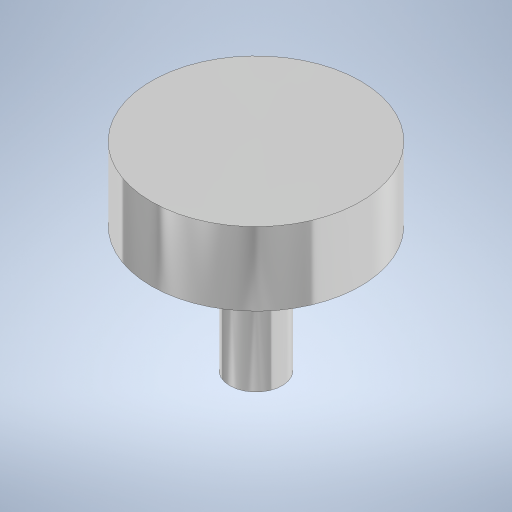
# Autodesk Inventor part: micromanipulator_knob
Saved by Autodesk Inventor 2024 (Build 280153000, 153)
## iProperties
Created: 2023-06-14
Part Number: micromanipulator_knob
Material: Generic
Document SubType Name: Modeling
Designer: dsdan
Density: 1 g/cm^3
Appearance: Chrome - Polished
Author: dsdan
Autodesk Inventor part; units mm, degrees
ref_plane "YZ Plane" through (0, 0, 0) normal (1, 0, 0) x (0, 1, 0)
ref_plane "XZ Plane" through (0, 0, 0) normal (0, 1, 0) x (-1, 0, 0)
ref_plane "XY Plane" through (0, 0, 0) normal (0, 0, 1) x (1, 0, 0)
sketch "Sketch1" plane through (0, 0, 0) normal (1, 0, 0) x (0, 1, 0)
  line L0 (-7.75, 2.5) -> (7.75, 2.5)
  line L1 (7.75, 2.5) -> (7.75, -2.5)
  line L2 (7.75, -2.5) -> (-7.75, -2.5)
  line L3 (-7.75, -2.5) -> (-7.75, 2.5)
  line L4 (-7.75, 2.5) -> (7.75, -2.5) construction
  line L5 (7.75, 2.5) -> (-7.75, -2.5) construction
  line L6 (11.25, 10) -> (4.25, 10)
  line L7 (4.25, 10) -> (4.25, -10)
  line L8 (4.25, -10) -> (11.25, -10)
  line L9 (11.25, -10) -> (11.25, 10)
  line L10 (11.25, 10) -> (4.25, -10) construction
  line L11 (4.25, 10) -> (11.25, -10) construction
  line L12 (-7.75, 0) -> (11.25, 0)
  point P0 (0, 0)
  point P1 (7.75, 0)
  point P2 (4.25, 2.5)
  dimension "d0" = 5
  dimension "d1" = 20
  dimension "d2" = 7
  dimension "d3" = 12
  constraints: 26 end point, 7 midpoint, 4 parallel, 2 horizontal, 2 perpendicular
  measures "d0" distance of L2.end L0.start
  measures "d1" distance of L8.end L6.start
  measures "d2" distance of L6.start L6.end
  measures "d3" distance between parallel lines of L3 L7
revolve "Revolution1" add sketch "Sketch1" angle 360 about axis through (0, -7.75, 0) along (0, 1, 0) contours L0 L7 L12 L3 | L7 L6 L9 L12 L1 L0 | L0 L1 L12 L7
body "Solid1"
